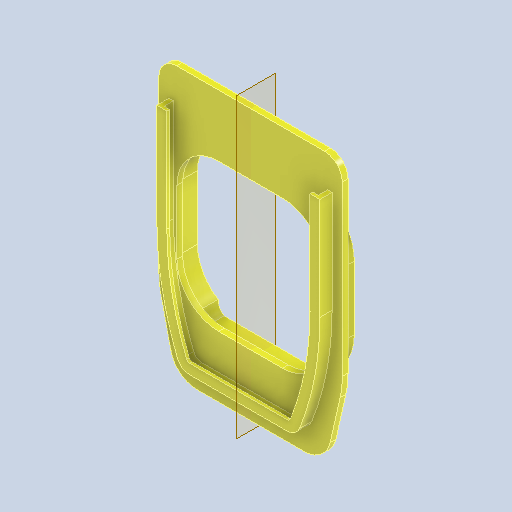
# Autodesk Inventor part: daVinciTool_Aufnahme
Saved by Autodesk Inventor 2024 (Build 280153000, 153)
## iProperties
Created: 2022-08-11
Part Number: daVinciTool_Aufnahme
Material: PMMA-Kunststoff
Document SubType Name: Modeling
Designer: alexw
Density: 1.188 g/cm^3
Appearance: Gelb
Mass: 27.4469 g
Surface Area: 208.635 cm^2
Volume: 23.1035 cm^3
Author: alexw
Autodesk Inventor part; units mm, degrees
ref_plane "YZ Plane" through (0, 0, 0) normal (1, 0, 0) x (0, 1, 0)
ref_plane "XZ Plane" through (0, 0, 0) normal (0, 1, 0) x (-1, 0, 0)
ref_plane "XY Plane" through (0, 0, 0) normal (0, 0, 1) x (1, 0, 0)
sketch "Skizze1" plane through (0, 0, 0) normal (0, 0, 1) x (1, 0, 0)
  line L0 (-33.4, 0) -> (33.4, 0)
  line L1 (41.4, -8) -> (41.4, -84.0456)
  line L2 (40.4201, -92.8453) -> (35.956, -112.6399)
  line L3 (24.25, -122) -> (-24.25, -122)
  line L4 (-35.956, -112.6399) -> (-40.4201, -92.8453)
  line L5 (-41.4, -84.0456) -> (-41.4, -8)
  line L6 (0, 0) -> (0, -122) construction
  arc A0 (-41.4, -84.0456) -> (-40.4201, -92.8453) centre (-1.4, -84.0456) ccw
  arc A1 (40.4201, -92.8453) -> (41.4, -84.0456) centre (1.4, -84.0456) ccw
  arc A2 (-35.956, -112.6399) -> (-24.25, -122) centre (-24.25, -110) ccw
  arc A3 (24.25, -122) -> (35.956, -112.6399) centre (24.25, -110) ccw
  arc A4 (-33.4, 0) -> (-41.4, -8) centre (-33.4, -8) ccw
  arc A5 (41.4, -8) -> (33.4, 0) centre (33.4, -8) ccw
  point P0 (33.8452, -122)
  point P1 (-33.8452, -122)
  point P2 (-41.4, -88.5)
  dimension "d1" = 82.8
  dimension "d2" = 122
  dimension "d3" = 33.5
  dimension "d4" = 40
  dimension "d5" = 12
  dimension "d6" = 8
  dimension "d15" = 48.5
  constraints: 14 end point, 12 point on circle, 12 tangent, 6 centre point, 6 point on line, 3 equal radius, 2 midpoint, 2 parallel, 1 coincident, 1 equal length, 1 horizontal, 1 perpendicular, 1 vertical
  measures "d1" distance between parallel lines of L1 L5
  measures "d2" distance between parallel lines of L0 L3
  measures "d3" distance from line of L3 point (-41.4, -88.5)
  measures "d4" radius of A0
  measures "d5" radius of A2
  measures "d6" radius of A4
  measures "d15" distance of L3.start L3.end
extrude "Extrusion1" add sketch "Skizze1" along normal blind 2.6
sketch "Skizze2" plane through (0, 0, 2.6) normal (0, 0, 1) x (1, 0, 0)
  line L0 (-36.8, -14.4) -> (-36.8, -60.5202)
  arc A0 (-36.8, -60.5202) -> (-27.5742, -108.62) centre (93.2, -60.5202) ccw
  line L1 (-22, -112.4) -> (22, -112.4)
  line L2 (36.8, -14.4) -> (36.8, -60.5202)
  arc A1 (27.5742, -108.62) -> (36.8, -60.5202) centre (-93.2, -60.5202) ccw
  line L3 (-36.8, -60.5202) -> (36.8, -60.5202) construction
  line L4 (-36.8, -14.4) -> (36.8, -14.4) construction
  line L5 (0, 0) -> (0, -122) construction
  line L6 (-24.25, -122) -> (24.25, -122) construction
  arc A2 (-27.5742, -108.62) -> (-22, -112.4) centre (-22, -106.4) ccw
  arc A3 (22, -112.4) -> (27.5742, -108.62) centre (22, -106.4) ccw
  line L7 (41.4, -84.0456) -> (41.4, -8) construction
  line L8 (-41.4, -8) -> (-41.4, -84.0456) construction
  line L9 (-34.8, -60.5202) -> (-34.8, -14.4)
  line L10 (34.8, -14.4) -> (34.8, -60.5202)
  arc A4 (25.7161, -107.88) -> (34.8, -60.5202) centre (-93.2, -60.5202) ccw
  arc A5 (22, -110.4) -> (25.7161, -107.88) centre (22, -106.4) ccw
  line L11 (22, -110.4) -> (-22, -110.4)
  arc A6 (-25.7161, -107.88) -> (-22, -110.4) centre (-22, -106.4) ccw
  arc A7 (-34.8, -60.5202) -> (-25.7161, -107.88) centre (93.2, -60.5202) ccw
  line L12 (-36.8, -14.4) -> (-34.8, -14.4)
  line L13 (34.8, -14.4) -> (36.8, -14.4)
  point P0 (-25.9993, -112.4)
  point P1 (25.9993, -112.4)
  point P2 (0, -14.4)
  dimension "d9" = 6
  dimension "d10" = 6
  dimension "d11" = 130
  dimension "d12" = 4.6
  dimension "d13" = 9.6
  dimension "d14" = 44
  dimension "d16" = 14.4
  dimension "d17" = 2
  constraints: 22 end point, 18 point on circle, 8 centre point, 7 tangent, 5 point on line, 2 collinear, 2 horizontal, 2 midpoint, 2 perpendicular, 2 vertical, 1 equal radius, 5 other
  measures "d9" radius of A2
  measures "d10" radius of A3
  measures "d11" radius of A0
  measures "d12" distance between parallel lines of L2 L7
  measures "d13" distance between parallel lines of L1 L6
  measures "d14" distance of L1.end L1.start
  measures "d16" distance from line of L5.start L4
  measures "d17" distance between parallel lines of L0 L9
extrude "Extrusion2" add sketch "Skizze2" along normal blind 5.5
sketch "Skizze3" plane through (-36.8, -14.4, 2.6) normal (0, 1, 0) x (1, 0, 0)
  line L0 (2, -4.2) -> (4.5, -4.2)
  line L1 (4.5, -4.2) -> (4.5, -5.5)
  line L2 (4.5, -5.5) -> (2, -5.5)
  line L3 (2, -5.5) -> (2, -4.2)
  line L4 (0, 0) -> (0, -5.5) projected
  point P0 (36.8, 2.6)
  dimension "d20" = 4.5
  dimension "d21" = 1.3
  constraints: 8 end point, 2 parallel, 1 coincident, 1 horizontal, 1 perpendicular
  measures "d20" distance between parallel lines of L1 L4
  measures "d21" distance between parallel lines of L0 L2
sketch "Skizze4" plane through (0, 0, 8.1) normal (0, 0, 1) x (1, 0, 0)
  line L0 (-34.8, -60.5202) -> (-34.8, -14.4) projected
  arc A0 (-34.8, -60.5202) -> (-25.7161, -107.88) centre (93.2, -60.5202) ccw projected
  arc A1 (-25.7161, -107.88) -> (-22, -110.4) centre (-22, -106.4) ccw projected
  line L1 (22, -110.4) -> (-22, -110.4) projected
  arc A2 (22, -110.4) -> (25.7161, -107.88) centre (22, -106.4) ccw projected
  arc A3 (25.7161, -107.88) -> (34.8, -60.5202) centre (-93.2, -60.5202) ccw projected
  line L2 (34.8, -14.4) -> (34.8, -60.5202) projected
  point P0 (0, 0)
sketch3d "3D-Skizze1"
  line L0 (-34.8, -14.4, 8.1) -> (-34.8, -60.5202, 8.1)
  arc A0 (-34.8, -60.5202, 8.1) -> (-25.7161, -107.88, 8.1) centre (93.2, -60.5202, 8.1) ccw
  arc A1 (-25.7161, -107.88, 8.1) -> (-22, -110.4, 8.1) centre (-22, -106.4, 8.1) ccw
  line L1 (-22, -110.4, 8.1) -> (22, -110.4, 8.1)
  arc A2 (22, -110.4, 8.1) -> (25.7161, -107.88, 8.1) centre (22, -106.4, 8.1) ccw
  arc A3 (25.7161, -107.88, 8.1) -> (34.8, -60.5202, 8.1) centre (-93.2, -60.5202, 8.1) ccw
  line L2 (34.8, -60.5202, 8.1) -> (34.8, -14.4, 8.1)
sweep "Sweeping1" add profiles "Skizze3" path "3D-Skizze1"
sketch "Skizze5" plane through (0, 0, 0) normal (0, 0, -1) x (-1, 0, 0)
  line L0 (-36.4, -24.7) -> (36.4, -24.7)
  line L1 (36.4, -24.7) -> (36.4, -97.5)
  line L2 (36.4, -97.5) -> (-36.4, -97.5)
  line L3 (-36.4, -97.5) -> (-36.4, -24.7)
  line L4 (-36.4, -24.7) -> (36.4, -97.5) construction
  line L5 (36.4, -24.7) -> (-36.4, -97.5) construction
  circle A0 centre (14.4, -46.7) radius 22 construction
  line L6 (0, 0) -> (0, -122) construction
  line L7 (24.25, -122) -> (-24.25, -122) construction
  line L8 (34.4, -26.7) -> (-34.4, -26.7)
  line L9 (-34.4, -26.7) -> (-34.4, -95.5)
  line L10 (-34.4, -95.5) -> (34.4, -95.5)
  line L11 (34.4, -95.5) -> (34.4, -26.7)
  line L12 (34.4, -26.7) -> (-34.4, -95.5) construction
  line L13 (-34.4, -26.7) -> (34.4, -95.5) construction
  circle A1 centre (-14.4, -46.7) radius 22 construction
  circle A2 centre (-14.4, -75.5) radius 22 construction
  circle A3 centre (14.4, -75.5) radius 22 construction
  line L14 (41.4, -8) -> (41.4, -84.0456) construction
  arc A4 (-36.4, -75.5) -> (-14.4, -97.5) centre (-14.4, -75.5) ccw
  arc A5 (-14.4, -24.7) -> (-36.4, -46.7) centre (-14.4, -46.7) ccw
  arc A6 (36.4, -46.7) -> (14.4, -24.7) centre (14.4, -46.7) ccw
  arc A7 (14.4, -97.5) -> (36.4, -75.5) centre (14.4, -75.5) ccw
  line L15 (-25.3, -97.5) -> (-19.1, -97.5)
  line L16 (-19.1, -97.5) -> (-19.1, -108)
  line L17 (-19.1, -108) -> (-25.3, -108)
  line L18 (-25.3, -108) -> (-25.3, -97.5)
  line L19 (19.1, -97.5) -> (25.3, -97.5)
  line L20 (25.3, -97.5) -> (25.3, -108)
  line L21 (25.3, -108) -> (19.1, -108)
  line L22 (19.1, -108) -> (19.1, -97.5)
  line L23 (-19.1, -108) -> (19.1, -108) construction
  arc A8 (-14.4, -26.7) -> (-34.4, -46.7) centre (-14.4, -46.7) ccw
  arc A9 (34.4, -46.7) -> (14.4, -26.7) centre (14.4, -46.7) ccw
  arc A10 (14.4, -95.5) -> (34.4, -75.5) centre (14.4, -75.5) ccw
  arc A11 (-34.4, -75.5) -> (-14.4, -95.5) centre (-14.4, -75.5) ccw
  line L24 (-25.3, -97.5) -> (-31.9034, -88.8279)
  line L25 (25.3, -97.5) -> (31.9034, -88.8279)
  line L26 (-19.1, -98.5) -> (19.1, -98.5)
  line L27 (19.1, -98.5) -> (19.1, -99.7)
  line L28 (19.1, -99.7) -> (-19.1, -99.7)
  line L29 (-19.1, -99.7) -> (-19.1, -98.5)
  arc A12 (-25.0991, -92.3976) -> (-19.1, -98.5) centre (-19.1, -92.5) ccw
  arc A13 (19.1, -98.5) -> (25.0991, -92.3976) centre (19.1, -92.5) ccw
  line L30 (-31.55, -16) -> (-25.45, -16)
  line L31 (-25.45, -16) -> (-25.45, -25.8)
  line L32 (-25.45, -25.8) -> (-31.55, -25.8)
  line L33 (-31.55, -25.8) -> (-31.55, -16)
  line L34 (25.45, -16) -> (31.55, -16)
  line L35 (31.55, -16) -> (31.55, -25.8)
  line L36 (31.55, -25.8) -> (25.45, -25.8)
  line L37 (25.45, -25.8) -> (25.45, -16)
  line L38 (-25.45, -16) -> (25.45, -16) construction
  line L39 (-29.75, -25.8) -> (-31.5142, -32.876)
  line L40 (29.75, -25.8) -> (31.5142, -32.876)
  line L41 (-29.75, -25.8) -> (-29.75, -30.94) construction
  line L42 (29.75, -25.8) -> (29.75, -30.94) construction
  line L43 (-25.45, -25.8) -> (-25.45, -30.0297)
  line L44 (25.45, -25.8) -> (25.45, -30.0297)
  line L45 (-33.25, -27.85) -> (33.25, -27.85)
  line L46 (33.25, -27.85) -> (33.25, -94.35)
  line L47 (33.25, -94.35) -> (-33.25, -94.35)
  line L48 (-33.25, -94.35) -> (-33.25, -27.85)
  line L49 (-33.25, -27.85) -> (33.25, -94.35) construction
  line L50 (33.25, -27.85) -> (-33.25, -94.35) construction
  circle A14 centre (-14.4, -75.5) radius 18.85
  circle A15 centre (-14.4, -46.7) radius 18.85
  circle A16 centre (14.4, -46.7) radius 18.85
  circle A17 centre (14.4, -75.5) radius 18.85
  point P0 (0, -61.1)
  point P1 (0, -24.7)
  point P2 (0, -108)
  point P3 (0, -16)
  point P4 (34.4, -46.7)
  point P5 (34.4, -75.5)
  point P6 (22.4166, -97.5)
  point P7 (-22.4166, -97.5)
  point P8 (-34.4, -75.5)
  point P9 (-34.4, -46.7)
  point P10 (-33.25, -40.0159)
  point P11 (-33.25, -82.1841)
  point P12 (-21.0841, -94.35)
  point P13 (21.0841, -94.35)
  point P14 (33.25, -82.1841)
  point P15 (33.25, -40.0159)
  point P16 (21.0841, -27.85)
  point P17 (-21.0841, -27.85)
  point P18 (14.4, -27.85)
  point P19 (-14.4, -27.85)
  point P20 (-33.25, -46.7)
  point P21 (-33.25, -75.5)
  point P22 (-14.4, -94.35)
  point P23 (14.4, -94.35)
  point P24 (33.25, -75.5)
  point P25 (33.25, -46.7)
  dimension "d25" = 2
  dimension "d26" = 22
  dimension "d27" = 5
  dimension "d29" = 6.2
  dimension "d30" = 6.2
  dimension "d31" = 38.2
  dimension "d33" = 1.2
  dimension "d34" = 3
  dimension "d35" = 6
  dimension "d36" = 6
  dimension "d37" = 63.1
  dimension "d38" = 6.1
  dimension "d39" = 6.1
  dimension "d40" = 92
  dimension "d41" = 9.8
  dimension "d42" = 37.287
  dimension "d44" = 1.8
  dimension "d45" = 1.8
  dimension "d46" = 14
  dimension "d79" = 66.5
  dimension "d80" = 66.5
  dimension "d83" = 22.3
  dimension "d84" = 14
  constraints: 98 end point, 38 point on circle, 26 point on line, 18 centre point, 17 parallel, 17 tangent, 10 midpoint, 10 perpendicular, 8 horizontal, 7 equal radius, 4 coincident, 4 concentric, 3 vertical, 1 collinear, 1 equal length
  measures "d25" distance between parallel lines of L3 L9
  measures "d26" radius of A0
  measures "d27" distance between parallel lines of L14 L1
  measures "d29" distance between parallel lines of L16 L18
  measures "d30" distance between parallel lines of L20 L22
  measures "d31" distance between parallel lines of L22 L16
  measures "d33" distance between parallel lines of L28 L26
  measures "d34" distance between parallel lines of L10 L26
  measures "d35" radius of A12
  measures "d36" radius of A13
  measures "d37" distance between parallel lines of L35 L33
  measures "d38" distance between parallel lines of L31 L33
  measures "d39" distance between parallel lines of L37 L35
  measures "d40" distance between parallel lines of L38 L23
  measures "d41" distance between parallel lines of L30 L32
  measures "d42" angle of L24 L18
  measures "d44" distance of L32.end L39.start
  measures "d45" distance of L35.end L40.start
  measures "d46" angle of L41 L39
  measures "d79" distance between parallel lines of L46 L48
  measures "d80" distance between parallel lines of L45 L47
  measures "d83" distance between parallel lines of L28 L7
  measures "d84" distance between parallel lines of L21 L7
extrude "Extrusion3" add sketch "Skizze5" along normal blind 7.8 contours L31 L32 L33 L0 | L0 L33 L30 L31 | L37 L34 L35 L0 | L0 L35 L36 L37 | L43 L8 L39 L32 | L43 A5 L45 L39 L8 | L43 L45 A5 | L36 L40 L8 L44 | L8 L40 L45 A6 L44 | A6 L45 L44 | L45 L43 A8 L48 A5 | A5 L39 L45 | L45 L40 A6 | A6 L46 A9 L44 L45 | A5 L9 A4 L3 | L1 A7 L11 A6 | A5 L48 A8 L9 | L11 A9 L46 A6 | L9 A11 L48 A4 | A7 L46 A10 L11 | L24 L10 A12 L2 | L2 A12 L16 L17 L18 | L48 A11 A12 L47 A4 | L20 L21 L22 A13 L2 | L2 A13 L10 L25 | A7 L47 A13 A10 L46 | L2 L16 A12 | L24 L47 A4 A12 L10 | A4 L47 L24 | A13 L22 L2 | L10 A13 A7 L47 L25 | L25 L47 A7 | L2 L22 L26 L16 | L26 L22 L28 L16 | L47 A12 A4 | A7 A13 L47
sketch "Skizze6" plane through (31.55, -25.8, 0) normal (1, 0, 0) x (0, 0, -1)
  line L0 (0, 0) -> (7.8, 0) construction
  circle A0 centre (4.15, 5.05) radius 1.55
  line L1 (7.8, 9.8) -> (7.8, 0) projected
  line L2 (4.15, 3.5) -> (7.8, 3.5)
  line L3 (4.15, 6.6) -> (7.8, 6.6)
  line L4 (2.6, 5.05) -> (2.6, 0) construction
  circle A1 centre (4.15, -76.95) radius 1.55
  line L5 (2.6, -76.95) -> (2.6, -82.2)
  line L6 (0, -82.2) -> (7.8, -82.2) construction
  line L7 (2.6, -82.2) -> (5.7, -82.2)
  line L8 (5.7, -82.2) -> (5.7, -76.95)
  line L9 (4.15, -75.4) -> (7.8, -75.4) construction
  line L10 (7.8, -71.7) -> (7.8, -82.2) construction
  line L11 (4.15, -82.2) -> (4.15, -76.95) construction
  line L12 (7.8, -20.9) -> (7.8, -49.7) construction
  line L13 (4.15, 5.05) -> (4.15, -76.95) construction
  point P0 (0, 25.8)
  dimension "d49" = 3.1
  dimension "d50" = 3.5
  dimension "d76" = 6.8
  dimension "d77" = 3.1
  dimension "d78" = 5.2
  constraints: 18 end point, 6 point on circle, 5 perpendicular, 5 tangent, 4 point on line, 2 centre point, 2 collinear, 2 horizontal, 1 midpoint, 1 vertical
  measures "d49" diameter of A0
  measures "d50" distance between parallel lines of L0 L2
  measures "d76" distance between parallel lines of L6 L9
  measures "d77" diameter of A1
  measures "d78" distance between parallel lines of L10 L5
extrude "Extrusion4" cut sketch "Skizze6" against normal through all
ref_plane "Arbeitsebene1" through (0, -75.5, 0) normal (1, 0, 0) x (0, 0, -1)
extrude "Extrusion5" cut sketch "Skizze5" against normal up to surface (2.6 mm away) contours L45 A16 A15 | A15 A16 A14 | A16 A17 A15 | A15 A16 | A15 A14 L48 | L46 A17 A16 | A16 A17 A14 A15 | A14 A15 A17 | A14 A15 | A17 A14 A16 | A16 A17 | A14 A17 L47 | A14 A17
equation "\"d9\" = d10"
equation "\"d30\" = d29"
equation "\"d36\" = d35"
